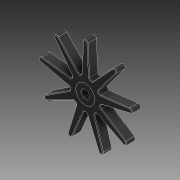
# Autodesk Inventor part: Simple Wheel Generator
Saved by Autodesk Inventor 2023 (Build 270158000, 158)
## iProperties
Created: 2022-01-26
Material: Rubber
Document SubType Name: Modeling
Designer: Desktop
Density: 0.93 g/cm^3
Appearance: Rubber - Black
Author: Desktop
Autodesk Inventor part; units mm, degrees
ref_plane "YZ Plane" through (0, 0, 0) normal (1, 0, 0) x (0, 1, 0)
ref_plane "XZ Plane" through (0, 0, 0) normal (0, 1, 0) x (-1, 0, 0)
ref_plane "XY Plane" through (0, 0, 0) normal (0, 0, 1) x (1, 0, 0)
sketch "Sketch1" plane through (0, 0, 0) normal (0, 0, 1) x (1, 0, 0)
  circle A0 centre (0, 0) radius 12.7
  line L0 (-6.3791, 0) -> (-3.1896, 5.5245)
  line L1 (-3.1896, 5.5245) -> (3.1896, 5.5245)
  line L2 (3.1896, 5.5245) -> (6.3791, 0)
  line L3 (6.3791, 0) -> (3.1896, -5.5245)
  line L4 (3.1896, -5.5245) -> (-3.1896, -5.5245)
  line L5 (-3.1896, -5.5245) -> (-6.3791, 0)
  circle A1 centre (0, 0) radius 63.5 construction
  line L6 (-2.9958, 60.6593) -> (-5.054, 21.9572)
  line L7 (2.9958, 60.6593) -> (5.054, 21.9572)
  arc A2 (2.9958, 60.6593) -> (-2.9958, 60.6593) centre (0, 60.5) ccw
  arc A3 (-10.2422, 20.0688) -> (-5.054, 21.9572) centre (-8.0498, 22.1165) ccw
  arc A4 (-36.6962, 48.3934) -> (-41.2859, 44.5421) centre (-38.8887, 46.3457) ccw
  line L8 (-36.6962, 48.3934) -> (-10.2422, 20.0688)
  line L9 (-41.2859, 44.5421) -> (-17.9854, 13.5715)
  arc A5 (-20.746, 8.79) -> (-17.9854, 13.5715) centre (-20.3827, 11.768) ccw
  arc A6 (-59.2176, 13.4836) -> (-60.258, 7.5831) centre (-59.5809, 10.5057) ccw
  line L10 (-59.2176, 13.4836) -> (-20.746, 8.79)
  line L11 (-60.258, 7.5831) -> (-22.5012, -1.1644)
  arc A7 (-21.5425, -6.6017) -> (-22.5012, -1.1644) centre (-23.1783, -4.087) ccw
  arc A8 (-54.0304, -27.7352) -> (-51.0346, -32.9241) centre (-52.3945, -30.25) ccw
  line L12 (-54.0304, -27.7352) -> (-21.5425, -6.6017)
  line L13 (-51.0346, -32.9241) -> (-16.4885, -15.3555)
  arc A9 (-12.259, -18.9044) -> (-16.4885, -15.3555) centre (-15.1286, -18.0295) ccw
  arc A10 (-23.5618, -55.9765) -> (-17.9316, -58.0257) centre (-20.6922, -56.8514) ccw
  line L14 (-23.5618, -55.9765) -> (-12.259, -18.9044)
  line L15 (-17.9316, -58.0257) -> (-2.7606, -22.3616)
  arc A11 (2.7606, -22.3616) -> (-2.7606, -22.3616) centre (0, -23.5359) ccw
  arc A12 (17.9316, -58.0257) -> (23.5618, -55.9765) centre (20.6922, -56.8514) ccw
  line L16 (17.9316, -58.0257) -> (2.7606, -22.3616)
  line L17 (23.5618, -55.9765) -> (12.259, -18.9044)
  arc A13 (16.4885, -15.3555) -> (12.259, -18.9044) centre (15.1286, -18.0295) ccw
  arc A14 (51.0346, -32.9241) -> (54.0304, -27.7352) centre (52.3945, -30.25) ccw
  line L18 (51.0346, -32.9241) -> (16.4885, -15.3555)
  line L19 (54.0304, -27.7352) -> (21.5425, -6.6017)
  arc A15 (22.5012, -1.1644) -> (21.5425, -6.6017) centre (23.1783, -4.087) ccw
  arc A16 (60.258, 7.5831) -> (59.2176, 13.4836) centre (59.5809, 10.5057) ccw
  line L20 (60.258, 7.5831) -> (22.5012, -1.1644)
  line L21 (59.2176, 13.4836) -> (20.746, 8.79)
  arc A17 (17.9854, 13.5715) -> (20.746, 8.79) centre (20.3827, 11.768) ccw
  arc A18 (41.2859, 44.5421) -> (36.6962, 48.3934) centre (38.8887, 46.3457) ccw
  line L22 (41.2859, 44.5421) -> (17.9854, 13.5715)
  line L23 (36.6962, 48.3934) -> (10.2422, 20.0688)
  arc A19 (5.054, 21.9572) -> (10.2422, 20.0688) centre (8.0498, 22.1165) ccw
  line L24 (0, 0) -> (0, 70.6946) construction
  circle A20 centre (0, 0) radius 20.5359 construction
  circle A21 centre (0, 0) radius 15.9004
  circle A22 centre (0, 0) radius 15.875
  circle A23 centre (0, 0) radius 6.3791
  point P0 (-10.2422, 20.0688)
  point P1 (-20.746, 8.79)
  point P2 (-21.5425, -6.6017)
  point P3 (-12.259, -18.9044)
  point P4 (2.7606, -22.3616)
  point P5 (16.4885, -15.3555)
  point P6 (22.5012, -1.1644)
  point P7 (17.9854, 13.5715)
  dimension "d0" = 25.4
  dimension "d1" = 11.049
  dimension "d2" = 127
  dimension "d3" = 3
  dimension "d7" = 360
  dimension "d9" = 41.0718
  dimension "d15" = 0.0254
  dimension "d16" = 3.175
  dimension "d19" = 6.3209
  constraints: 50 end point, 36 point on circle, 23 centre point, 6 tangent, 5 coincident, 1 equal radius, 1 horizontal, 1 horizontal alignment, 1 vertical, 1 vertical alignment, 116 other
  measures "d0" diameter of A0
  measures "d1" distance between parallel lines of L4 L1
  measures "d2" diameter of A1
  measures "d3" radius of A2
  measures "d9" diameter of A20
  measures "d15" radial gap between concentric circles of A21 A22
  measures "d16" radial gap between concentric circles of A0 A22
extrude "Body" add sketch "Sketch1" along normal mid plane 12.7 contours A2 L7 A19 L23 A18 L22 A17 L21 A16 L20 A15 L19 A14 L18 A13 L17 A12 L16 A11 L15 A10 L14 A9 L13 A8 L12 A7 L11 A6 L10 A5 L9 A4 L8 A3 L6 | A21 | A22
fillet "Fillet1" radius 0.7937 72 edges at (4.0249, 41.3083, 6.35) (0, 63.5, 6.35) (-4.0249, 41.3083, 6.35) (-7.0237, 19.2974, 6.35) (-23.4692, 34.2311, 6.35) (-40.817, 48.6438, 6.35) (-29.6357, 29.0568, 6.35) (-17.7846, 10.268, 6.35) (-39.9818, 11.1368, 6.35) (-62.5353, 11.0267, 6.35) (-41.3796, 3.2094, 6.35) (-20.2239, -3.566, 6.35) (-37.7864, -17.1685, 6.35) (-54.9926, -31.75, 6.35) (-33.7616, -24.1398, 6.35) (-13.2002, -15.7314, 6.35) (-17.9104, -37.4405, 6.35) (-21.7183, -59.6705, 6.35) (-10.3461, -40.1937, 6.35) (0, -20.5359, 6.35) (10.3461, -40.1937, 6.35) (21.7183, -59.6705, 6.35) (17.9104, -37.4405, 6.35) (13.2002, -15.7314, 6.35) (33.7616, -24.1398, 6.35) (54.9926, -31.75, 6.35) (37.7864, -17.1685, 6.35) (20.2239, -3.566, 6.35) (41.3796, 3.2094, 6.35) (62.5353, 11.0267, 6.35) (39.9818, 11.1368, 6.35) (17.7846, 10.268, 6.35) (29.6357, 29.0568, 6.35) (40.817, 48.6438, 6.35) (23.4692, 34.2311, 6.35) (7.0237, 19.2974, 6.35) (39.9818, 11.1368, -6.35) (62.5353, 11.0267, -6.35) (41.3796, 3.2094, -6.35) (20.2239, -3.566, -6.35) (37.7864, -17.1685, -6.35) (54.9926, -31.75, -6.35) (33.7616, -24.1398, -6.35) (13.2002, -15.7314, -6.35) (17.9104, -37.4405, -6.35) (21.7183, -59.6705, -6.35) (10.3461, -40.1937, -6.35) (0, -20.5359, -6.35) (-10.3461, -40.1937, -6.35) (-21.7183, -59.6705, -6.35) (-17.9104, -37.4405, -6.35) (-13.2002, -15.7314, -6.35) (-33.7616, -24.1398, -6.35) (-54.9926, -31.75, -6.35) (-37.7864, -17.1685, -6.35) (-20.2239, -3.566, -6.35) (-41.3796, 3.2094, -6.35) (-62.5353, 11.0267, -6.35) (-39.9818, 11.1368, -6.35) (-17.7846, 10.268, -6.35) (-29.6357, 29.0568, -6.35) (-40.817, 48.6438, -6.35) (-23.4692, 34.2311, -6.35) (-7.0237, 19.2974, -6.35) (-4.0249, 41.3083, -6.35) (0, 63.5, -6.35) (4.0249, 41.3083, -6.35) (7.0237, 19.2974, -6.35) (23.4692, 34.2311, -6.35) (40.817, 48.6438, -6.35) (29.6357, 29.0568, -6.35) (17.7846, 10.268, -6.35)
extrude "Extrusion2" add sketch "Sketch1" along normal mid plane 12.7 separate body contours A0 | A23 L0 | L5 A23 | A23 L1 | L4 A23 | A23 L2 | L3 A23
body "Solid1"
body "Solid2"
